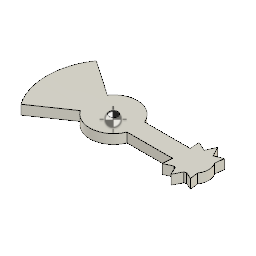
Good Morning... v2 (Autodesk Fusion 360 design; units mm, degrees)
Autodesk Fusion 360 part; units mm, degrees
note: some values were not read from the file. Chosen so that the rebuilt part matches the saved one: which face or edge a step refers to. Set by a fixed rule: which sketch regions a step uses.
sketch "Sketch1" plane through (0, 0, 0) normal (0, 0, 1) x (1, 0, 0)
  circle A0 centre (0, 0) radius 2.7
  circle A1 centre (0, 0) radius 15
  circle A2 centre (0, 0) radius 60
  line L0 (0, 5.5) -> (59.7474, 5.5)
  line L1 (0, 0) -> (60, 0) construction
  line L2 (0, -5.5) -> (59.7474, -5.5)
  circle A3 centre (50.5062, -0.3422) radius 9.5
  line L3 (59.0183, 10.8091) -> (53.8956, 8.5326)
  line L4 (58.3065, 5.0805) -> (59.0183, 10.8091)
  line L5 (53.8956, 8.5326) -> (58.3065, 5.0805)
  line L6 (50.6806, 14.6809) -> (47.9726, 8.8137)
  line L7 (53.8956, 8.5326) -> (50.6806, 14.6809)
  line L8 (49.5676, 8.4672) -> (53.8956, 8.5326)
  line L9 (42.1632, 11.5894) -> (42.5886, 4.9078)
  line L10 (47.9726, 8.8137) -> (42.1632, 11.5894)
  line L11 (44.3482, 5.8115) -> (47.9726, 8.8137)
  line L12 (53.8956, -8.5326) -> (58.3065, -5.0805)
  line L13 (58.3065, -5.0805) -> (59.0183, -10.8091)
  line L14 (59.0183, -10.8091) -> (53.8956, -8.5326)
  line L15 (50.6806, -14.6809) -> (47.9726, -8.8137)
  line L16 (53.8956, -8.5326) -> (50.6806, -14.6809)
  line L17 (49.5676, -8.4672) -> (53.8956, -8.5326)
  line L18 (42.1632, -11.5894) -> (42.5886, -4.9078)
  line L19 (47.9726, -8.8137) -> (42.1632, -11.5894)
  line L20 (44.3482, -5.8115) -> (47.9726, -8.8137)
  line L21 (0, 0) -> (-34.5316, 23.7329)
  line L22 (0, 0) -> (-34.5316, -23.7329)
  circle A4 centre (0, 0) radius 41.9008
  dimension "d1" = 5.4
  dimension "d2" = 30
  dimension "d3" = 120
  dimension "d4" = 5.5
  dimension "d7" = 145.5
  dimension "d8" = 19
  constraint coincident A0.centre A1.centre
  constraint coincident A2 L0.end
  constraint horizontal L0
  constraint coincident A2 L1.end
  constraint horizontal L1
  constraint symmetric L0.start L1 L2.start
  constraint symmetric L0.end L1 L2.end
  constraint coincident L1.end A3
  constraint symmetric L1 L4.start L12.end
  constraint symmetric L1 L3.start L13.end
  constraint symmetric L1 L3.end L12.start
  constraint symmetric L1 L6.start L15.start
  constraint symmetric L1 L6.end L15.end
  constraint symmetric L1 L8.start L17.start
  constraint symmetric L1 L9.start L18.start
  constraint symmetric L1 L9.end L18.end
  constraint symmetric L1 L11.start L20.start
  constraint symmetric L1 A0.centre A1.centre
  constraint symmetric L1 L21.end L22.end
  constraint concentric A2 A4
  constraint coincident L21.end A4
  constraint coincident A3 L9.end
  constraint coincident A3 L6.end
  constraint coincident A3 L3.end
  constraint coincident A3 L4.start
  constraint coincident A2 L3.start
  measures "d1" diameter of A0
  measures "d2" diameter of A1
  measures "d3" diameter of A2
  measures "d4" distance of L0 L1
  measures "d7" angle of L1 L21
  measures "d8" diameter of A3
extrude "Extrude1" add sketch "Sketch1" along normal mid plane 6 contours A0 A1 L21 L22 | A0 A1 L21 L22 | A1 L21 L22 A4 | A1 L0 L2 A3 A4 | L0 A3 L9 A4 | L2 A3 A4 | L0 A3 L9 L10 | L0 A3 L9 | A3 A4 | A2 L0 L2 A3 L5 L12 L13 A4 | L2 A3 L18 | L0 A3 L5 | L2 A3 L12 L15 L16 L18 L19 | A3 L18 L19 | L0 A3 L5 | L0 A3 L5 | A3 L6 L7 | L2 L12 L13 | L2 A3 L12 L13 L14 | A3 L15 L19 | L0 A3 L3 L4 | L0 A3 L4 | L2 A3 L13 | A3 L14 L16 | A3 L15 L16 | A2 A3 | A3 L13 L14
